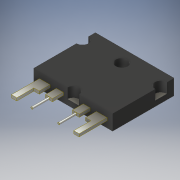
# Autodesk Inventor part: schunt
Saved by Autodesk Inventor 2017 (Build 210142000, 142)
## iProperties
Part Number: schunt
Material: Generisch
Document SubType Name: Modeling
Designer: Philomena-Theresa
Density: 1 g/cm^3
Appearance: Vorgabe
Author: Philomena-Theresa
Autodesk Inventor part; units mm, degrees
ref_plane "YZ Plane" through (0, 0, 0) normal (1, 0, 0) x (0, 1, 0)
ref_plane "XZ Plane" through (0, 0, 0) normal (0, 1, 0) x (-1, 0, 0)
ref_plane "XY Plane" through (0, 0, 0) normal (0, 0, 1) x (1, 0, 0)
sketch "Skizze1" plane through (0, 0, 0) normal (0, 0, 1) x (1, 0, 0)
  line L0 (-11.235, 8.775) -> (11.235, 8.775)
  line L1 (11.235, 8.775) -> (11.235, -8.775)
  line L2 (11.235, -8.775) -> (-11.235, -8.775)
  line L3 (-11.235, -8.775) -> (-11.235, 8.775)
  line L4 (-11.235, 8.775) -> (11.235, -8.775) construction
  point P0 (0, 0)
  point P1 (0, 0)
  dimension "d0" = 22.47
  dimension "d1" = 17.55
  constraints: 10 end point, 2 parallel, 1 coincident, 1 horizontal, 1 midpoint, 1 perpendicular
  measures "d0" distance of L1.end L2.end
  measures "d1" distance of L0.end L1.end
extrude "Extrusion1" add sketch "Skizze1" along normal blind 4.37
sketch "Skizze2" plane through (0, 0, 4.37) normal (0, 0, 1) x (1, 0, 0)
  line L0 (11.235, 8.775) -> (-11.235, 8.775) construction
  line L1 (-11.235, 8.775) -> (-11.235, 6.775) construction
  line L2 (-11.235, 8.775) -> (-11.235, -8.775) construction
  line L3 (-11.235, 6.775) -> (0, 6.775) construction
  line L4 (0, 6.775) -> (0, 5.075) construction
  circle A0 centre (0, 5.075) radius 1.7
  point P0 (0, 0)
  dimension "d4" = 2
  dimension "d5" = 1.7
  dimension "d6" = 3.4
  constraints: 6 end point, 2 perpendicular, 1 centre point, 1 coincident, 1 point on line
  measures "d4" distance of L0.end L1.end
  measures "d5" distance of L3.end L4.end
  measures "d6" diameter of A0
extrude "Extrusion2" cut sketch "Skizze2" against normal blind 4.37
sketch "Skizze4" plane through (0, 0, 4.37) normal (0, 0, 1) x (1, 0, 0)
  circle A0 centre (0, 5.075) radius 1.7 projected
  line L0 (-11.235, 8.775) -> (-11.235, -8.775) construction
  line L1 (-11.235, 5.075) -> (11.1798, 5.075) construction
  circle A1 centre (-11.235, 5.075) radius 1.7
  circle A2 centre (11.1798, 5.075) radius 1.7
  line L2 (-11.235, -8.775) -> (11.235, -8.775) construction
  circle A3 centre (0, -8.775) radius 1.7
  point P0 (0, 0)
  dimension "d14" = 3.4
  dimension "d15" = 3.4
  dimension "d16" = 3.4
  constraints: 3 centre point, 2 coincident, 2 end point, 1 horizontal, 1 midpoint, 1 point on line
  measures "d14" diameter of A1
  measures "d15" diameter of A2
  measures "d16" diameter of A3
extrude "Extrusion4" cut sketch "Skizze4" against normal blind 2.88 contours A1 | A2 | A3
sketch "Skizze5" plane through (-11.235, -8.775, 0) normal (0, -1, 0) x (1, 0, 0)
  line L0 (9.535, 1.49) -> (9.535, 4.37) projected
  line L1 (0, 4.37) -> (9.535, 4.37) projected
  line L2 (0, 0) -> (0, 4.37) projected
  line L3 (22.47, 0) -> (0, 0) projected
  line L4 (22.47, 0) -> (22.47, 4.37) projected
  line L5 (12.935, 4.37) -> (22.47, 4.37) projected
  line L6 (12.935, 4.37) -> (12.935, 1.49) projected
  line L7 (12.935, 1.49) -> (9.535, 1.49) projected
  line L8 (0, 0) -> (0, 4.37) projected
  line L9 (0, 2.185) -> (1.57, 2.185) construction
  line L10 (22.47, 0) -> (22.47, 4.37) projected
  line L11 (22.47, 2.185) -> (20.9, 2.185) construction
  line L12 (1.57, 2.585) -> (4.63, 2.585)
  line L13 (4.63, 2.585) -> (4.63, 1.785)
  line L14 (4.63, 1.785) -> (1.57, 1.785)
  line L15 (1.57, 1.785) -> (1.57, 2.585)
  line L16 (17.84, 2.585) -> (20.9, 2.585)
  line L17 (20.9, 2.585) -> (20.9, 1.785)
  line L18 (20.9, 1.785) -> (17.84, 1.785)
  line L19 (17.84, 1.785) -> (17.84, 2.585)
  point P0 (11.235, 0)
  dimension "d19" = 1.57
  dimension "d20" = 1.57
  dimension "d21" = 3.06
  dimension "d22" = 0.8
  dimension "d23" = 3.06
  dimension "d24" = 0.8
  constraints: 20 end point, 4 horizontal, 4 midpoint, 4 parallel, 2 perpendicular
  measures "d19" distance of L9.end L9.start
  measures "d20" distance of L11.end L11.start
  measures "d21" distance of L13.end L14.end
  measures "d22" distance of L12.end L13.end
  measures "d23" distance of L17.end L19.start
  measures "d24" distance of L17.start L17.end
extrude "Extrusion5" add sketch "Skizze5" along normal blind 8 separate body contours L12 L13 L14 L15 | L16 L17 L18 L19
sketch "Skizze6" plane through (-11.235, -16.775, 0) normal (0, -1, 0) x (1, 0, 0)
  line L0 (1.57, 1.785) -> (1.57, 2.585) construction
  line L1 (1.57, 2.185) -> (3.11, 2.185) construction
  line L2 (20.9, 1.785) -> (20.9, 2.585) construction
  line L3 (20.9, 2.185) -> (19.36, 2.185) construction
  line L4 (4.63, 2.585) -> (4.63, 1.785) projected
  line L5 (4.63, 2.585) -> (1.57, 2.585) projected
  line L6 (4.63, 1.785) -> (3.1, 1.785)
  line L7 (3.1, 1.785) -> (3.1, 2.585)
  line L8 (3.1, 2.585) -> (4.63, 2.585)
  line L9 (4.63, 2.585) -> (4.63, 1.785)
  line L10 (17.84, 2.585) -> (17.84, 1.785) projected
  line L11 (17.84, 1.785) -> (20.9, 1.785) projected
  line L12 (17.84, 2.585) -> (19.37, 2.585)
  line L13 (19.37, 2.585) -> (19.37, 1.785)
  line L14 (19.37, 1.785) -> (17.84, 1.785)
  line L15 (17.84, 1.785) -> (17.84, 2.585)
  point P0 (11.235, 0)
  dimension "d27" = 1.54
  dimension "d28" = 1.54
  constraints: 20 end point, 4 horizontal, 4 midpoint, 4 parallel, 2 perpendicular
  measures "d27" distance of L1.start L1.end
  measures "d28" distance of L3.start L3.end
extrude "Extrusion6" cut sketch "Skizze6" against normal blind 4.88 bodies 2
sketch "Skizze7" plane through (-11.235, -8.775, 0) normal (0, -1, 0) x (1, 0, 0)
  line L0 (4.63, 2.585) -> (4.63, 1.785) construction
  line L1 (4.63, 2.185) -> (6.39, 2.185) construction
  line L2 (17.84, 2.585) -> (17.84, 1.785) construction
  line L3 (17.84, 2.185) -> (16.08, 2.185) construction
  line L4 (6.39, 2.585) -> (8.39, 2.585)
  line L5 (8.39, 2.585) -> (8.39, 1.785)
  line L6 (8.39, 1.785) -> (6.39, 1.785)
  line L7 (6.39, 1.785) -> (6.39, 2.585)
  line L8 (14.08, 2.585) -> (16.08, 2.585)
  line L9 (16.08, 2.585) -> (16.08, 1.785)
  line L10 (16.08, 1.785) -> (14.08, 1.785)
  line L11 (14.08, 1.785) -> (14.08, 2.585)
  point P0 (11.235, 0)
  dimension "d31" = 1.76
  dimension "d32" = 1.76
  dimension "d33" = 2
  dimension "d34" = 0.8
  dimension "d35" = 2
  dimension "d36" = 0.8
  constraints: 20 end point, 4 horizontal, 4 midpoint, 4 parallel, 2 perpendicular
  measures "d31" distance of L1.end L1.start
  measures "d32" distance of L3.end L3.start
  measures "d33" distance of L5.end L6.end
  measures "d34" distance of L4.end L5.end
  measures "d35" distance of L9.end L10.end
  measures "d36" distance of L8.end L9.end
extrude "Extrusion7" add sketch "Skizze7" along normal blind 3.11 separate body
sketch "Skizze8" plane through (-11.235, -11.885, 0) normal (0, -1, 0) x (1, 0, 0)
  line L0 (8.39, 2.585) -> (6.39, 2.585) projected
  line L1 (6.39, 2.585) -> (6.39, 1.785) projected
  line L2 (6.39, 1.785) -> (8.39, 1.785) projected
  line L3 (8.39, 1.785) -> (8.39, 2.585) projected
  line L4 (16.08, 2.585) -> (14.08, 2.585) projected
  line L5 (14.08, 2.585) -> (14.08, 1.785) projected
  line L6 (14.08, 1.785) -> (16.08, 1.785) projected
  line L7 (16.08, 1.785) -> (16.08, 2.585) projected
  line L8 (6.39, 2.585) -> (8.39, 2.585) projected
  line L9 (8.39, 2.585) -> (8.39, 1.785) projected
  line L10 (6.39, 2.585) -> (8.39, 1.785) construction
  line L11 (16.08, 2.585) -> (14.08, 2.585) construction
  line L12 (14.08, 2.585) -> (16.08, 1.785) construction
  circle A0 centre (7.39, 2.185) radius 0.3
  circle A1 centre (15.08, 2.185) radius 0.3
  point P0 (11.235, 0)
  dimension "d39" = 0.6
  dimension "d40" = 0.6
  constraints: 4 end point, 2 centre point, 2 midpoint
  measures "d39" diameter of A0
  measures "d40" diameter of A1
extrude "Extrusion8" add sketch "Skizze8" along normal blind 4.88 contours A0 | A1 bodies 3
